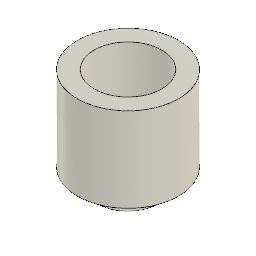
magnet-mounter-3.5-1.5 v6 (Autodesk Fusion 360 design; units mm, degrees)
Autodesk Fusion 360 part; units mm, degrees
sketch "スケッチ1" plane through (0, 0, 0) normal (0, 0, 1) x (1, 0, 0)
  circle A0 centre (0, 0) radius 0.5
  circle A1 centre (0, 0) radius 1
  circle A2 centre (0, 0) radius 1.5
  circle A3 centre (0, 0) radius 0.9
  dimension "d1" = 1
  dimension "d2" = 2
  dimension "d3" = 3
  dimension "d9" = 1.8
  measures "d1" diameter of A0
  measures "d2" diameter of A1
  measures "d3" diameter of A2
  measures "d9" diameter of A3
extrude "押し出し1" add sketch "スケッチ1" against normal blind 1 contours A3 makes body 1
extrude "押し出し2" add sketch "スケッチ1" along normal blind 2 separate body contours A2 makes body 2
extrude "押し出し3" add sketch "スケッチ1" against normal blind 0.5 contours A1 | A2 | A3 bodies 1 2
fillet "フィレット1" radius 1 1 edges at (-0.8391, 0.3255, -0.5) on bodies 1
